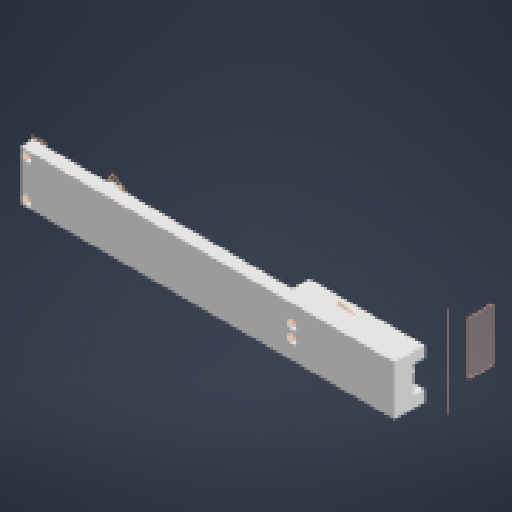
# Autodesk Inventor part: Secondary Rail
Saved by Autodesk Inventor 2025.2 (Build 292293000, 293)
## iProperties
Created: 2024-11-17
Part Number: Secondary Rail
Material: Generic
Document SubType Name: Modeling
Designer: JL
Density: 1 g/cm^3
Appearance: Default
Author: JL
Autodesk Inventor part; units mm, degrees
ref_plane "YZ Plane" through (0, 0, 0) normal (1, 0, 0) x (0, 1, 0)
ref_plane "Work Plane1" through (-111.4654, 31.6528, -127.3993) normal (0, 0, 1) x (0.9606716, -0.277687, 0)
ref_plane "Work Plane2" through (-75.2288, 52.4668, -179.3993) normal (1, 0, 0) x (0, 1, 0)
ref_plane "Work Plane3" through (-85.6621, 48.7987, -153.3993) normal (0, 0, 1) x (-0.8564988, 0.516149, 0)
sketch "Sketch1" plane through (-75.2288, 52.4668, -179.3993) normal (1, 0, 0) x (0, 1, 0)
  line L0 (10.9134, 26) -> (-63.0301, 26) projected
  line L1 (-40.35, -17.2) -> (-40.35, 7.5) construction
  line L2 (0.35, -17.2) -> (-40.35, -17.2) construction
  line L3 (0.35, -17.2) -> (0.35, 7.5) construction
  line L4 (-9, 7.5) -> (0.35, 7.5) construction
  line L5 (-9, -1) -> (-31, -1) construction
  line L6 (-40.35, 7.5) -> (-31, 7.5) construction
  line L7 (-40.35, 69.2) -> (-40.35, 44.5)
  line L8 (0.35, 69.2) -> (-40.35, 69.2)
  line L9 (0.35, 69.2) -> (0.35, 44.5)
  line L10 (-10, 44.5) -> (0.35, 44.5)
  line L11 (-10, 52) -> (-10, 44.5)
  line L12 (-30, 52) -> (-10, 52)
  line L13 (-30, 52) -> (-30, 44.5)
  line L14 (-40.35, 44.5) -> (-30, 44.5)
  line L15 (-9, 7.5) -> (-9, -1) projected
  line L16 (-31, -1) -> (-31, 7.5) projected
  point P0 (-52.4668, 179.3993)
  constraints: 16 end point, 4 symmetric about line
ref_plane "Work Plane6" through (-164.7503, 14.9668, -186.8993) normal (-1, 0, 0) x (0, 0, 1)
extrude "Extrusion2" add sketch "Sketch1" against normal up to surface (89.5216 mm away)
ref_plane "Work Plane7" through (-377.475, 32.4668, -120.7993) normal (0, 0, 1) x (1, 0, 0)
sketch "Sketch4" plane through (-377.475, 32.4668, -120.7993) normal (0, 0, 1) x (1, 0, 0)
  circle A0 centre (-0.0016, 15.35) radius 2.77 construction
  circle A1 centre (-0.0015, -15.3504) radius 2.77 construction
  line L0 (-5, -20.35) -> (5, -20.35) projected
  line L1 (5, -20.35) -> (5, 20.35) construction
  line L2 (5, 20.35) -> (-5, 20.35) projected
  line L3 (-5, 20.35) -> (-5, -20.35) projected
  line L4 (212.7246, 20.35) -> (212.7246, -20.35) projected
  line L5 (5, 20.35) -> (212.7246, 20.35)
  line L6 (212.7246, -20.35) -> (5, -20.35)
  point P0 (377.475, -32.4668)
  constraints: 4 end point, 2 perpendicular
extrude "Extrusion3" add sketch "Sketch4" along normal up to surface (10.6 mm away)
ref_plane "Work Plane8" through (-329.8595, 37.7187, -137.3993) normal (0, 0, 1) x (0.5075729, 0.8616088, 0)
sketch "Sketch5" plane through (-329.8595, 37.7187, -137.3993) normal (0, 0, 1) x (0.5075729, 0.8616088, 0)
  circle A0 centre (-6.0955, 0) radius 6.5 projected
  point P0 (134.929, -303.3548)
extrude "Extrusion4" add sketch "Sketch5" along normal up to next
sketch "Sketch6" plane through (-332.9534, 32.4668, -137.3993) normal (0, 0, -1) x (-1, 0, 0)
  circle A0 centre (0, 0) radius 2 projected
  point P0 (-332.9534, -32.4668)
ref_plane "Work Plane9" through (-338.8707, 26.0642, -143.3993) normal (0, 0, -1) x (0.5075729, 0.8616088, 0)
extrude "Extrusion5" add sketch "Sketch6" along normal up to surface (6 mm away) draft -2
sketch "Sketch7" plane through (-332.9534, 32.4668, -143.3993) normal (0, 0, -1) x (-1, 0, 0)
  circle A0 centre (0, 0) radius 1.7905 construction
  circle A1 centre (0, 0) radius 1.7905 construction
  circle A2 centre (-1.7905, 0) radius 0.2
  point P0 (-332.9534, -32.4668)
  dimension "d18" = 0.4
  constraints: 2 horizontal alignment, 1 centre point, 1 other
  measures "d18" diameter of A2
extrude "Extrusion6" add sketch "Sketch7" against normal up to next
pattern_circular "Circular Pattern1" count 6 over 360 about axis through (-332.9534, 32.4668, -137.3993) along (0, 0, -1) of "Extrusion6"
sketch "Sketch8" plane through (-377.475, 32.4668, -120.7993) normal (0, 0, -1) x (-1, 0, 0)
  line L0 (-212.7246, -20.35) -> (-212.7246, 20.35) projected
  line L1 (-207.7246, -20.35) -> (-207.7246, 20.35)
  line L2 (-212.7246, -20.35) -> (-207.7246, -20.35)
  line L3 (5, -20.35) -> (-212.7246, -20.35) projected
  line L4 (-212.7246, 20.35) -> (-207.7246, 20.35)
  point P0 (-377.475, -32.4668)
  dimension "d24" = 5
  constraints: 6 end point, 1 collinear, 1 parallel, 1 perpendicular
  measures "d24" distance between parallel lines of L0 L1
extrude "Extrusion7" add sketch "Sketch8" along normal up to surface (14.1 mm away)
sketch "Sketch3" plane through (-75.2288, 12.1168, -110.1993) normal (0, 0, 1) x (1, 0, 0)
  point P0 (75.2288, -12.1168)
  point P1 (-84.5216, 25.35)
  point P2 (-84.5216, 15.35)
  point P3 (-302.2462, 35.7)
  point P4 (-302.2462, 5)
hole "Hole1" at (-159.7503, 37.4668, -110.1993) at (-159.7503, 27.4668, -110.1993) at (-377.475, 17.1168, -110.1993) at (-377.475, 47.8168, -110.1993) direction (0, 0, -1) diameter 4.3 end through all counterbore diameter 8 counterbore depth 4 clearance for "Socket Head Cap Screw" size "M4" standard "Ansi Metric M Profile"
thicken "Thicken1" operation cut thickness 1 both sides no extend neighbours no toward (0, 1, 0) faces at (-134.9098, 42.4668, -132.3993) (-102.6912, 34.0471, -127.3993) (-134.9098, 22.4668, -132.3993) (-164.7503, 35.8001, -132.3993)
body "Solid2"
